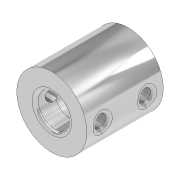
# Autodesk Inventor part: 5mm Coupler
Saved by Autodesk Inventor 2020 (Build 240168000, 168)
## iProperties
Created: 2021-06-28
Part Number: 5mm Coupler
Material: Generic
Document SubType Name: Modeling
Designer: Coy
Density: 1 g/cm^3
Appearance: Chrome - Polished
Author: Coy
Autodesk Inventor part; units mm, degrees
ref_plane "YZ Plane" through (0, 0, 0) normal (1, 0, 0) x (0, 1, 0)
ref_plane "XZ Plane" through (0, 0, 0) normal (0, 1, 0) x (-1, 0, 0)
ref_plane "XY Plane" through (0, 0, 0) normal (0, 0, 1) x (1, 0, 0)
sketch "Sketch1" plane through (0, 0, 0) normal (0, 0, 1) x (1, 0, 0)
  circle A0 centre (0, 0) radius 2.5
  circle A1 centre (0, 0) radius 4
  circle A2 centre (0, 0) radius 5.5
  dimension "d0" = 5
  dimension "d1" = 8
  dimension "d17" = 3
  constraints: 3 centre point, 2 coincident
  measures "d0" diameter of A0
  measures "d1" diameter of A1
  measures "d17" radial gap between concentric circles of A0 A2
extrude "Extrusion1" add sketch "Sketch1" along normal blind 12 contours A1 | A2
sketch "Sketch2" plane through (0, 0, 0) normal (1, 0, 0) x (0, 1, 0)
  line L0 (4, 12) -> (-4, 12) projected
  line L1 (4, 0) -> (-4, 0) projected
  line L2 (0, 12) -> (0, 7) construction
  line L3 (0, 0) -> (0, 5) construction
  circle A0 centre (0, 9.5) radius 1
  circle A1 centre (0, 2.5) radius 1
  dimension "d4" = 5
  dimension "d5" = 5
  dimension "d6" = 2
  dimension "d7" = 2
  constraints: 4 end point, 3 midpoint, 2 centre point, 2 vertical
  measures "d4" distance of L2.start L2.end
  measures "d5" distance of L3.start L3.end
  measures "d6" diameter of A0
  measures "d7" diameter of A1
extrude "Extrusion2" cut sketch "Sketch2" against normal through all both and the other way through all
chamfer "Chamfer1" distance 3 angle 2 1 edges at (-2.5, 0, 12) measured on face at (-2.5, 0, 11.5)
chamfer "Chamfer2" distance 3 angle 2 1 edges at (-2.5, 0, 0) measured on face at (-2.5, 0, 0.5)
fillet "Fillet1" radius 0.5 10 edges at (-2.6048, 0, 0) (-2.6048, 0, 12) (5.4496, 0.7429, 10.1693) (5.4083, -1, 9.5001) (5.4497, 0.7421, 8.8297) (5.4496, 0.7429, 3.1693) (5.4083, -1, 2.5001) (5.4497, 0.7421, 1.8297) (-5.4083, -1, 9.5056) (-5.4083, -1, 2.5056)
body "Solid1"
